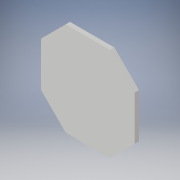
# Autodesk Inventor part: chassis
Saved by Autodesk Inventor 2018 (Build 220112000, 112)
## iProperties
Created: 2018-04-14
Part Number: chassis
Material: Generic
Document SubType Name: Modeling
Designer: dvyen
Density: 1 g/cm^3
Appearance: Default
Author: dvyen
Autodesk Inventor part; units mm, degrees
ref_plane "YZ Plane" through (0, 0, 0) normal (1, 0, 0) x (0, 1, 0)
ref_plane "XZ Plane" through (0, 0, 0) normal (0, 1, 0) x (-1, 0, 0)
ref_plane "XY Plane" through (0, 0, 0) normal (0, 0, 1) x (1, 0, 0)
sketch "Sketch3" plane through (0, 0, 0) normal (0, 0, 1) x (1, 0, 0)
  line L0 (-32, 32) -> (32, 32)
  line L1 (32, 32) -> (32, -32)
  line L2 (32, -32) -> (-32, -32)
  line L3 (-32, -32) -> (-32, 32)
  line L4 (-32, 32) -> (32, -32) construction
  line L5 (32, 32) -> (-32, -32) construction
  line L6 (-32, 32) -> (-15.171, 32)
  line L7 (-15.171, 32) -> (-15.171, 15.171)
  line L8 (-15.171, 15.171) -> (-32, 15.171)
  line L9 (-32, 15.171) -> (-32, 32)
  line L10 (-15.171, 32) -> (-32, 15.171)
  line L11 (32, 32) -> (15.171, 32)
  line L12 (15.171, 32) -> (15.171, 15.171)
  line L13 (15.171, 15.171) -> (32, 15.171)
  line L14 (32, 15.171) -> (32, 32)
  line L15 (15.171, 32) -> (32, 15.171)
  line L16 (-32, -32) -> (-15.171, -32)
  line L17 (-15.171, -32) -> (-15.171, -15.171)
  line L18 (-15.171, -15.171) -> (-32, -15.171)
  line L19 (-32, -15.171) -> (-32, -32)
  line L20 (32, -32) -> (15.171, -32)
  line L21 (15.171, -32) -> (15.171, -15.171)
  line L22 (15.171, -15.171) -> (32, -15.171)
  line L23 (32, -15.171) -> (32, -32)
  line L24 (-32, -15.171) -> (-15.171, -32)
  line L25 (32, -15.171) -> (15.171, -32)
  point P0 (0, 0)
  dimension "d21" = 64
  dimension "d22" = 64
  dimension "d23" = 16.829
  dimension "d24" = 16.829
  dimension "d25" = 16.829
  dimension "d26" = 16.829
  dimension "d27" = 16.829
  dimension "d28" = 16.829
  dimension "d29" = 16.829
  dimension "d30" = 16.829
  constraints: 52 end point, 10 parallel, 5 horizontal, 5 perpendicular, 2 midpoint
  measures "d21" distance of L1.end L2.end
  measures "d22" distance of L0.end L1.end
  measures "d23" distance of L7.end L8.end
  measures "d24" distance of L6.end L7.end
  measures "d25" distance of L13.end L12.end
  measures "d26" distance of L12.end L11.end
  measures "d27" distance of L18.end L17.end
  measures "d28" distance of L17.end L16.end
  measures "d29" distance of L21.end L22.end
  measures "d30" distance of L20.end L21.end
extrude "Extrusion3" add sketch "Sketch3" along normal blind 3 contours L0 L12 L13 L1 L22 L21 L2 L17 L18 L3 L8 L7 | L7 L8 L10 | L15 L13 L12 | L18 L17 L24 | L25 L21 L22
body "Solid2"
